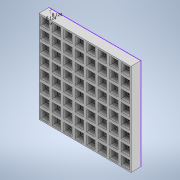
# Autodesk Inventor part: StandMatrix
Saved by Autodesk Inventor 2020.1 (Build 241239000, 239)
## iProperties
Created: 2019-09-02
Part Number: StandMatrix
Material: Generic
Document SubType Name: Modeling
Designer: matteo.spadetto-1
Density: 1 g/cm^3
Appearance: Default
Author: matteo.spadetto-1
Autodesk Inventor part; units mm, degrees
ref_plane "YZ Plane" through (0, 0, 0) normal (1, 0, 0) x (0, 1, 0)
ref_plane "XZ Plane" through (0, 0, 0) normal (0, 1, 0) x (-1, 0, 0)
ref_plane "XY Plane" through (0, 0, 0) normal (0, 0, 1) x (1, 0, 0)
sketch "Sketch1" plane through (0, 0, 0) normal (0, 0, 1) x (1, 0, 0)
  line L0 (1.062, 57.938) -> (1.062, 63.938)
  line L1 (1.062, 63.938) -> (7.062, 63.938)
  line L2 (7.062, 63.938) -> (7.062, 57.938)
  line L3 (7.062, 57.938) -> (1.062, 57.938)
  line L4 (17.31, 57.938) -> (23.31, 57.938)
  line L5 (23.31, 57.938) -> (23.31, 63.938)
  line L6 (23.31, 63.938) -> (17.31, 63.938)
  line L7 (17.31, 63.938) -> (17.31, 57.938)
  line L8 (9.186, 57.938) -> (15.186, 57.938)
  line L9 (15.186, 57.938) -> (15.186, 63.938)
  line L10 (15.186, 63.938) -> (9.186, 63.938)
  line L11 (9.186, 63.938) -> (9.186, 57.938)
  line L12 (25.434, 57.938) -> (31.434, 57.938)
  line L13 (31.434, 57.938) -> (31.434, 63.938)
  line L14 (31.434, 63.938) -> (25.434, 63.938)
  line L15 (25.434, 63.938) -> (25.434, 57.938)
  line L16 (33.558, 57.938) -> (39.558, 57.938)
  line L17 (39.558, 57.938) -> (39.558, 63.938)
  line L18 (39.558, 63.938) -> (33.558, 63.938)
  line L19 (33.558, 63.938) -> (33.558, 57.938)
  line L20 (47.682, 57.938) -> (41.682, 57.938)
  line L21 (41.682, 57.938) -> (41.682, 63.938)
  line L22 (41.682, 63.938) -> (47.682, 63.938)
  line L23 (47.682, 63.938) -> (47.682, 57.938)
  line L24 (55.806, 57.938) -> (49.806, 57.938)
  line L25 (49.806, 57.938) -> (49.806, 63.938)
  line L26 (49.806, 63.938) -> (55.806, 63.938)
  line L27 (55.806, 63.938) -> (55.806, 57.938)
  line L28 (63.93, 57.938) -> (57.93, 57.938)
  line L29 (57.93, 57.938) -> (57.93, 63.938)
  line L30 (57.93, 63.938) -> (63.93, 63.938)
  line L31 (63.93, 63.938) -> (63.93, 57.938)
  line L32 (1.062, 49.814) -> (1.062, 55.814)
  line L33 (1.062, 55.814) -> (7.062, 55.814)
  line L34 (7.062, 55.814) -> (7.062, 49.814)
  line L35 (7.062, 49.814) -> (1.062, 49.814)
  line L36 (9.186, 49.814) -> (15.186, 49.814)
  line L37 (15.186, 49.814) -> (15.186, 55.814)
  line L38 (15.186, 55.814) -> (9.186, 55.814)
  line L39 (9.186, 55.814) -> (9.186, 49.814)
  line L40 (17.31, 49.814) -> (17.31, 55.814)
  line L41 (17.31, 55.814) -> (23.31, 55.814)
  line L42 (23.31, 55.814) -> (23.31, 49.814)
  line L43 (23.31, 49.814) -> (17.31, 49.814)
  line L44 (25.434, 55.814) -> (31.434, 55.814)
  line L45 (31.434, 55.814) -> (31.434, 49.814)
  line L46 (31.434, 49.814) -> (25.434, 49.814)
  line L47 (33.558, 55.814) -> (39.558, 55.814)
  line L48 (39.558, 55.814) -> (39.558, 49.814)
  line L49 (39.558, 49.814) -> (33.558, 49.814)
  line L50 (47.682, 49.814) -> (41.682, 49.814)
  line L51 (41.682, 49.814) -> (41.682, 55.814)
  line L52 (41.682, 55.814) -> (47.682, 55.814)
  line L53 (47.682, 55.814) -> (47.682, 49.814)
  line L54 (49.806, 49.814) -> (55.806, 49.814)
  line L55 (55.806, 49.814) -> (55.806, 55.814)
  line L56 (55.806, 55.814) -> (49.806, 55.814)
  line L57 (49.806, 55.814) -> (49.806, 49.814)
  line L58 (63.93, 49.814) -> (57.93, 49.814)
  line L59 (57.93, 49.814) -> (57.93, 55.814)
  line L60 (57.93, 55.814) -> (63.93, 55.814)
  line L61 (63.93, 55.814) -> (63.93, 49.814)
  line L62 (1.062, 41.69) -> (7.062, 41.69)
  line L63 (7.062, 41.69) -> (7.062, 47.69)
  line L64 (7.062, 47.69) -> (1.062, 47.69)
  line L65 (1.062, 47.69) -> (1.062, 41.69)
  line L66 (9.186, 41.69) -> (9.186, 47.69)
  line L67 (9.186, 47.69) -> (15.186, 47.69)
  line L68 (15.186, 47.69) -> (15.186, 41.69)
  line L69 (15.186, 41.69) -> (9.186, 41.69)
  line L70 (23.31, 41.69) -> (23.31, 47.69)
  line L71 (23.31, 47.69) -> (17.31, 47.69)
  line L72 (17.31, 47.69) -> (17.31, 41.69)
  line L73 (17.31, 41.69) -> (23.31, 41.69)
  line L74 (31.434, 41.69) -> (25.434, 41.69)
  line L75 (25.434, 41.69) -> (25.434, 47.69)
  line L76 (25.434, 47.69) -> (31.434, 47.69)
  line L77 (31.434, 47.69) -> (31.434, 41.69)
  line L78 (39.558, 41.69) -> (33.558, 41.69)
  line L79 (33.558, 41.69) -> (33.558, 47.69)
  line L80 (33.558, 47.69) -> (39.558, 47.69)
  line L81 (39.558, 47.69) -> (39.558, 41.69)
  line L82 (47.682, 41.69) -> (47.682, 47.69)
  line L83 (47.682, 47.69) -> (41.682, 47.69)
  line L84 (41.682, 47.69) -> (41.682, 41.69)
  line L85 (41.682, 41.69) -> (47.682, 41.69)
  line L86 (55.806, 41.69) -> (55.806, 47.69)
  line L87 (55.806, 47.69) -> (49.806, 47.69)
  line L88 (49.806, 47.69) -> (49.806, 41.69)
  line L89 (49.806, 41.69) -> (55.806, 41.69)
  line L90 (63.93, 41.69) -> (63.93, 47.69)
  line L91 (63.93, 47.69) -> (57.93, 47.69)
  line L92 (57.93, 47.69) -> (57.93, 41.69)
  line L93 (57.93, 41.69) -> (63.93, 41.69)
  line L94 (7.062, 33.566) -> (1.062, 33.566)
  line L95 (1.062, 33.566) -> (1.062, 39.566)
  line L96 (1.062, 39.566) -> (7.062, 39.566)
  line L97 (7.062, 39.566) -> (7.062, 33.566)
  line L98 (15.186, 33.566) -> (15.186, 39.566)
  line L99 (15.186, 39.566) -> (9.186, 39.566)
  line L100 (9.186, 39.566) -> (9.186, 33.566)
  line L101 (9.186, 33.566) -> (15.186, 33.566)
  line L102 (17.31, 33.566) -> (23.31, 33.566)
  line L103 (23.31, 33.566) -> (23.31, 39.566)
  line L104 (23.31, 39.566) -> (17.31, 39.566)
  line L105 (17.31, 39.566) -> (17.31, 33.566)
  line L106 (25.434, 33.566) -> (31.434, 33.566)
  line L107 (31.434, 33.566) -> (31.434, 39.566)
  line L108 (31.434, 39.566) -> (25.434, 39.566)
  line L109 (25.434, 39.566) -> (25.434, 33.566)
  line L110 (39.558, 33.566) -> (33.558, 33.566)
  line L111 (33.558, 33.566) -> (33.558, 39.566)
  line L112 (33.558, 39.566) -> (39.558, 39.566)
  line L113 (39.558, 39.566) -> (39.558, 33.566)
  line L114 (41.682, 33.566) -> (41.682, 39.566)
  line L115 (41.682, 39.566) -> (47.682, 39.566)
  line L116 (47.682, 39.566) -> (47.682, 33.566)
  line L117 (47.682, 33.566) -> (41.682, 33.566)
  line L118 (55.806, 33.566) -> (49.806, 33.566)
  line L119 (49.806, 33.566) -> (49.806, 39.566)
  line L120 (49.806, 39.566) -> (55.806, 39.566)
  line L121 (55.806, 39.566) -> (55.806, 33.566)
  line L122 (63.93, 33.566) -> (57.93, 33.566)
  line L123 (57.93, 33.566) -> (57.93, 39.566)
  line L124 (57.93, 39.566) -> (63.93, 39.566)
  line L125 (63.93, 39.566) -> (63.93, 33.566)
  line L126 (25.434, 49.814) -> (25.434, 55.814)
  line L127 (33.558, 55.814) -> (33.558, 49.814)
  line L128 (1.062, 7.062) -> (1.062, 1.062)
  line L129 (1.062, 1.062) -> (7.062, 1.062)
  line L130 (7.062, 1.062) -> (7.062, 7.062)
  line L131 (7.062, 7.062) -> (1.062, 7.062)
  line L132 (17.31, 7.062) -> (23.31, 7.062)
  line L133 (23.31, 7.062) -> (23.31, 1.062)
  line L134 (23.31, 1.062) -> (17.31, 1.062)
  line L135 (17.31, 1.062) -> (17.31, 7.062)
  line L136 (9.186, 7.062) -> (15.186, 7.062)
  line L137 (15.186, 7.062) -> (15.186, 1.062)
  line L138 (15.186, 1.062) -> (9.186, 1.062)
  line L139 (9.186, 1.062) -> (9.186, 7.062)
  line L140 (25.434, 7.062) -> (31.434, 7.062)
  line L141 (31.434, 7.062) -> (31.434, 1.062)
  line L142 (31.434, 1.062) -> (25.434, 1.062)
  line L143 (25.434, 1.062) -> (25.434, 7.062)
  line L144 (33.558, 7.062) -> (39.558, 7.062)
  line L145 (39.558, 7.062) -> (39.558, 1.062)
  line L146 (39.558, 1.062) -> (33.558, 1.062)
  line L147 (33.558, 1.062) -> (33.558, 7.062)
  line L148 (47.682, 7.062) -> (41.682, 7.062)
  line L149 (41.682, 7.062) -> (41.682, 1.062)
  line L150 (41.682, 1.062) -> (47.682, 1.062)
  line L151 (47.682, 1.062) -> (47.682, 7.062)
  line L152 (55.806, 7.062) -> (49.806, 7.062)
  line L153 (49.806, 7.062) -> (49.806, 1.062)
  line L154 (49.806, 1.062) -> (55.806, 1.062)
  line L155 (55.806, 1.062) -> (55.806, 7.062)
  line L156 (63.93, 7.062) -> (57.93, 7.062)
  line L157 (57.93, 7.062) -> (57.93, 1.062)
  line L158 (57.93, 1.062) -> (63.93, 1.062)
  line L159 (63.93, 1.062) -> (63.93, 7.062)
  line L160 (1.062, 15.186) -> (1.062, 9.186)
  line L161 (1.062, 9.186) -> (7.062, 9.186)
  line L162 (7.062, 9.186) -> (7.062, 15.186)
  line L163 (7.062, 15.186) -> (1.062, 15.186)
  line L164 (9.186, 15.186) -> (15.186, 15.186)
  line L165 (15.186, 15.186) -> (15.186, 9.186)
  line L166 (15.186, 9.186) -> (9.186, 9.186)
  line L167 (9.186, 9.186) -> (9.186, 15.186)
  line L168 (17.31, 15.186) -> (17.31, 9.186)
  line L169 (17.31, 9.186) -> (23.31, 9.186)
  line L170 (23.31, 9.186) -> (23.31, 15.186)
  line L171 (23.31, 15.186) -> (17.31, 15.186)
  line L172 (25.434, 9.186) -> (31.434, 9.186)
  line L173 (31.434, 9.186) -> (31.434, 15.186)
  line L174 (31.434, 15.186) -> (25.434, 15.186)
  line L175 (33.558, 9.186) -> (39.558, 9.186)
  line L176 (39.558, 9.186) -> (39.558, 15.186)
  line L177 (39.558, 15.186) -> (33.558, 15.186)
  line L178 (47.682, 15.186) -> (41.682, 15.186)
  line L179 (41.682, 15.186) -> (41.682, 9.186)
  line L180 (41.682, 9.186) -> (47.682, 9.186)
  line L181 (47.682, 9.186) -> (47.682, 15.186)
  line L182 (49.806, 15.186) -> (55.806, 15.186)
  line L183 (55.806, 15.186) -> (55.806, 9.186)
  line L184 (55.806, 9.186) -> (49.806, 9.186)
  line L185 (49.806, 9.186) -> (49.806, 15.186)
  line L186 (63.93, 15.186) -> (57.93, 15.186)
  line L187 (57.93, 15.186) -> (57.93, 9.186)
  line L188 (57.93, 9.186) -> (63.93, 9.186)
  line L189 (63.93, 9.186) -> (63.93, 15.186)
  line L190 (1.062, 23.31) -> (7.062, 23.31)
  line L191 (7.062, 23.31) -> (7.062, 17.31)
  line L192 (7.062, 17.31) -> (1.062, 17.31)
  line L193 (1.062, 17.31) -> (1.062, 23.31)
  line L194 (9.186, 23.31) -> (9.186, 17.31)
  line L195 (9.186, 17.31) -> (15.186, 17.31)
  line L196 (15.186, 17.31) -> (15.186, 23.31)
  line L197 (15.186, 23.31) -> (9.186, 23.31)
  line L198 (23.31, 23.31) -> (23.31, 17.31)
  line L199 (23.31, 17.31) -> (17.31, 17.31)
  line L200 (17.31, 17.31) -> (17.31, 23.31)
  line L201 (17.31, 23.31) -> (23.31, 23.31)
  line L202 (31.434, 23.31) -> (25.434, 23.31)
  line L203 (25.434, 23.31) -> (25.434, 17.31)
  line L204 (25.434, 17.31) -> (31.434, 17.31)
  line L205 (31.434, 17.31) -> (31.434, 23.31)
  line L206 (39.558, 23.31) -> (33.558, 23.31)
  line L207 (33.558, 23.31) -> (33.558, 17.31)
  line L208 (33.558, 17.31) -> (39.558, 17.31)
  line L209 (39.558, 17.31) -> (39.558, 23.31)
  line L210 (47.682, 23.31) -> (47.682, 17.31)
  line L211 (47.682, 17.31) -> (41.682, 17.31)
  line L212 (41.682, 17.31) -> (41.682, 23.31)
  line L213 (41.682, 23.31) -> (47.682, 23.31)
  line L214 (55.806, 23.31) -> (55.806, 17.31)
  line L215 (55.806, 17.31) -> (49.806, 17.31)
  line L216 (49.806, 17.31) -> (49.806, 23.31)
  line L217 (49.806, 23.31) -> (55.806, 23.31)
  line L218 (63.93, 23.31) -> (63.93, 17.31)
  line L219 (63.93, 17.31) -> (57.93, 17.31)
  line L220 (57.93, 17.31) -> (57.93, 23.31)
  line L221 (57.93, 23.31) -> (63.93, 23.31)
  line L222 (7.062, 31.434) -> (1.062, 31.434)
  line L223 (1.062, 31.434) -> (1.062, 25.434)
  line L224 (1.062, 25.434) -> (7.062, 25.434)
  line L225 (7.062, 25.434) -> (7.062, 31.434)
  line L226 (15.186, 31.434) -> (15.186, 25.434)
  line L227 (15.186, 25.434) -> (9.186, 25.434)
  line L228 (9.186, 25.434) -> (9.186, 31.434)
  line L229 (9.186, 31.434) -> (15.186, 31.434)
  line L230 (17.31, 31.434) -> (23.31, 31.434)
  line L231 (23.31, 31.434) -> (23.31, 25.434)
  line L232 (23.31, 25.434) -> (17.31, 25.434)
  line L233 (17.31, 25.434) -> (17.31, 31.434)
  line L234 (25.434, 31.434) -> (31.434, 31.434)
  line L235 (31.434, 31.434) -> (31.434, 25.434)
  line L236 (31.434, 25.434) -> (25.434, 25.434)
  line L237 (25.434, 25.434) -> (25.434, 31.434)
  line L238 (39.558, 31.434) -> (33.558, 31.434)
  line L239 (33.558, 31.434) -> (33.558, 25.434)
  line L240 (33.558, 25.434) -> (39.558, 25.434)
  line L241 (39.558, 25.434) -> (39.558, 31.434)
  line L242 (41.682, 31.434) -> (41.682, 25.434)
  line L243 (41.682, 25.434) -> (47.682, 25.434)
  line L244 (47.682, 25.434) -> (47.682, 31.434)
  line L245 (47.682, 31.434) -> (41.682, 31.434)
  line L246 (55.806, 31.434) -> (49.806, 31.434)
  line L247 (49.806, 31.434) -> (49.806, 25.434)
  line L248 (49.806, 25.434) -> (55.806, 25.434)
  line L249 (55.806, 25.434) -> (55.806, 31.434)
  line L250 (63.93, 31.434) -> (57.93, 31.434)
  line L251 (57.93, 31.434) -> (57.93, 25.434)
  line L252 (57.93, 25.434) -> (63.93, 25.434)
  line L253 (63.93, 25.434) -> (63.93, 31.434)
  line L254 (25.434, 15.186) -> (25.434, 9.186)
  line L255 (33.558, 9.186) -> (33.558, 15.186)
  line L256 (0, 65) -> (0, 0)
  line L257 (0, 0) -> (65, 0)
  line L258 (0, 65) -> (65, 65)
  line L259 (65, 65) -> (65, 0)
  line L260 (6.562, 63.438) -> (6.562, 58.438)
  line L261 (6.562, 58.438) -> (1.562, 58.438)
  line L262 (1.562, 58.438) -> (1.562, 63.438)
  line L263 (1.562, 63.438) -> (6.562, 63.438)
  line L264 (9.686, 63.438) -> (14.686, 63.438)
  line L265 (14.686, 63.438) -> (14.686, 58.438)
  line L266 (14.686, 58.438) -> (9.686, 58.438)
  line L267 (9.686, 58.438) -> (9.686, 63.438)
  line L268 (17.81, 63.438) -> (22.81, 63.438)
  line L269 (22.81, 63.438) -> (22.81, 58.438)
  line L270 (22.81, 58.438) -> (17.81, 58.438)
  line L271 (17.81, 58.438) -> (17.81, 63.438)
  line L272 (25.934, 63.438) -> (30.934, 63.438)
  line L273 (30.934, 63.438) -> (30.934, 58.438)
  line L274 (30.934, 58.438) -> (25.934, 58.438)
  line L275 (25.934, 58.438) -> (25.934, 63.438)
  line L276 (34.058, 63.438) -> (39.058, 63.438)
  line L277 (39.058, 63.438) -> (39.058, 58.438)
  line L278 (39.058, 58.438) -> (34.058, 58.438)
  line L279 (34.058, 58.438) -> (34.058, 63.438)
  line L280 (42.182, 63.438) -> (47.182, 63.438)
  line L281 (47.182, 63.438) -> (47.182, 58.438)
  line L282 (47.182, 58.438) -> (42.182, 58.438)
  line L283 (42.182, 58.438) -> (42.182, 63.438)
  line L284 (50.306, 63.438) -> (55.306, 63.438)
  line L285 (55.306, 63.438) -> (55.306, 58.438)
  line L286 (55.306, 58.438) -> (50.306, 58.438)
  line L287 (50.306, 58.438) -> (50.306, 63.438)
  line L288 (58.43, 63.438) -> (63.43, 63.438)
  line L289 (63.43, 63.438) -> (63.43, 58.438)
  line L290 (63.43, 58.438) -> (58.43, 58.438)
  line L291 (58.43, 58.438) -> (58.43, 63.438)
  line L292 (1.562, 55.314) -> (6.562, 55.314)
  line L293 (6.562, 55.314) -> (6.562, 50.314)
  line L294 (6.562, 50.314) -> (1.562, 50.314)
  line L295 (1.562, 50.314) -> (1.562, 55.314)
  line L296 (9.686, 55.314) -> (14.686, 55.314)
  line L297 (14.686, 55.314) -> (14.686, 50.314)
  line L298 (14.686, 50.314) -> (9.686, 50.314)
  line L299 (9.686, 50.314) -> (9.686, 55.314)
  line L300 (17.81, 55.314) -> (22.81, 55.314)
  line L301 (22.81, 55.314) -> (22.81, 50.314)
  line L302 (22.81, 50.314) -> (17.81, 50.314)
  line L303 (17.81, 50.314) -> (17.81, 55.314)
  line L304 (25.934, 55.314) -> (30.934, 55.314)
  line L305 (30.934, 55.314) -> (30.934, 50.314)
  line L306 (30.934, 50.314) -> (25.934, 50.314)
  line L307 (25.934, 50.314) -> (25.934, 55.314)
  line L308 (34.058, 55.314) -> (39.058, 55.314)
  line L309 (39.058, 55.314) -> (39.058, 50.314)
  line L310 (39.058, 50.314) -> (34.058, 50.314)
  line L311 (34.058, 50.314) -> (34.058, 55.314)
  line L312 (42.182, 55.314) -> (47.182, 55.314)
  line L313 (47.182, 55.314) -> (47.182, 50.314)
  line L314 (47.182, 50.314) -> (42.182, 50.314)
  line L315 (42.182, 50.314) -> (42.182, 55.314)
  line L316 (50.306, 55.314) -> (55.306, 55.314)
  line L317 (55.306, 55.314) -> (55.306, 50.314)
  line L318 (55.306, 50.314) -> (50.306, 50.314)
  line L319 (50.306, 50.314) -> (50.306, 55.314)
  line L320 (58.43, 55.314) -> (63.43, 55.314)
  line L321 (63.43, 55.314) -> (63.43, 50.314)
  line L322 (63.43, 50.314) -> (58.43, 50.314)
  line L323 (58.43, 50.314) -> (58.43, 55.314)
  line L324 (1.562, 47.19) -> (6.562, 47.19)
  line L325 (6.562, 47.19) -> (6.562, 42.19)
  line L326 (6.562, 42.19) -> (1.562, 42.19)
  line L327 (1.562, 42.19) -> (1.562, 47.19)
  line L328 (9.686, 47.19) -> (14.686, 47.19)
  line L329 (14.686, 47.19) -> (14.686, 42.19)
  line L330 (14.686, 42.19) -> (9.686, 42.19)
  line L331 (9.686, 42.19) -> (9.686, 47.19)
  line L332 (17.81, 47.19) -> (22.81, 47.19)
  line L333 (22.81, 47.19) -> (22.81, 42.19)
  line L334 (22.81, 42.19) -> (17.81, 42.19)
  line L335 (17.81, 42.19) -> (17.81, 47.19)
  line L336 (25.934, 47.19) -> (30.934, 47.19)
  line L337 (30.934, 47.19) -> (30.934, 42.19)
  line L338 (30.934, 42.19) -> (25.934, 42.19)
  line L339 (25.934, 42.19) -> (25.934, 47.19)
  line L340 (34.058, 47.19) -> (39.058, 47.19)
  line L341 (39.058, 47.19) -> (39.058, 42.19)
  line L342 (39.058, 42.19) -> (34.058, 42.19)
  line L343 (34.058, 42.19) -> (34.058, 47.19)
  line L344 (42.182, 47.19) -> (47.182, 47.19)
  line L345 (47.182, 47.19) -> (47.182, 42.19)
  line L346 (47.182, 42.19) -> (42.182, 42.19)
  line L347 (42.182, 42.19) -> (42.182, 47.19)
  line L348 (50.306, 47.19) -> (55.306, 47.19)
  line L349 (55.306, 47.19) -> (55.306, 42.19)
  line L350 (55.306, 42.19) -> (50.306, 42.19)
  line L351 (50.306, 42.19) -> (50.306, 47.19)
  line L352 (58.43, 47.19) -> (63.43, 47.19)
  line L353 (63.43, 47.19) -> (63.43, 42.19)
  line L354 (63.43, 42.19) -> (58.43, 42.19)
  line L355 (58.43, 42.19) -> (58.43, 47.19)
  line L356 (1.562, 39.066) -> (6.562, 39.066)
  line L357 (6.562, 39.066) -> (6.562, 34.066)
  line L358 (6.562, 34.066) -> (1.562, 34.066)
  line L359 (1.562, 34.066) -> (1.562, 39.066)
  line L360 (9.686, 39.066) -> (14.686, 39.066)
  line L361 (14.686, 39.066) -> (14.686, 34.066)
  line L362 (14.686, 34.066) -> (9.686, 34.066)
  line L363 (9.686, 34.066) -> (9.686, 39.066)
  line L364 (17.81, 39.066) -> (22.81, 39.066)
  line L365 (22.81, 39.066) -> (22.81, 34.066)
  line L366 (22.81, 34.066) -> (17.81, 34.066)
  line L367 (17.81, 34.066) -> (17.81, 39.066)
  line L368 (25.934, 39.066) -> (30.934, 39.066)
  line L369 (30.934, 39.066) -> (30.934, 34.066)
  line L370 (30.934, 34.066) -> (25.934, 34.066)
  line L371 (25.934, 34.066) -> (25.934, 39.066)
  line L372 (34.058, 39.066) -> (39.058, 39.066)
  line L373 (39.058, 39.066) -> (39.058, 34.066)
  line L374 (39.058, 34.066) -> (34.058, 34.066)
  line L375 (34.058, 34.066) -> (34.058, 39.066)
  line L376 (42.182, 39.066) -> (47.182, 39.066)
  line L377 (47.182, 39.066) -> (47.182, 34.066)
  line L378 (47.182, 34.066) -> (42.182, 34.066)
  line L379 (42.182, 34.066) -> (42.182, 39.066)
  line L380 (50.306, 39.066) -> (55.306, 39.066)
  line L381 (55.306, 39.066) -> (55.306, 34.066)
  line L382 (55.306, 34.066) -> (50.306, 34.066)
  line L383 (50.306, 34.066) -> (50.306, 39.066)
  line L384 (58.43, 39.066) -> (63.43, 39.066)
  line L385 (63.43, 39.066) -> (63.43, 34.066)
  line L386 (63.43, 34.066) -> (58.43, 34.066)
  line L387 (58.43, 34.066) -> (58.43, 39.066)
  line L388 (1.562, 30.942) -> (6.562, 30.942)
  line L389 (6.562, 30.942) -> (6.562, 25.942)
  line L390 (6.562, 25.942) -> (1.562, 25.942)
  line L391 (1.562, 25.942) -> (1.562, 30.942)
  line L392 (9.686, 30.942) -> (14.686, 30.942)
  line L393 (14.686, 30.942) -> (14.686, 25.942)
  line L394 (14.686, 25.942) -> (9.686, 25.942)
  line L395 (9.686, 25.942) -> (9.686, 30.942)
  line L396 (17.81, 30.942) -> (22.81, 30.942)
  line L397 (22.81, 30.942) -> (22.81, 25.942)
  line L398 (22.81, 25.942) -> (17.81, 25.942)
  line L399 (17.81, 25.942) -> (17.81, 30.942)
  line L400 (25.934, 30.942) -> (30.934, 30.942)
  line L401 (30.934, 30.942) -> (30.934, 25.942)
  line L402 (30.934, 25.942) -> (25.934, 25.942)
  line L403 (25.934, 25.942) -> (25.934, 30.942)
  line L404 (34.058, 30.942) -> (39.058, 30.942)
  line L405 (39.058, 30.942) -> (39.058, 25.942)
  line L406 (39.058, 25.942) -> (34.058, 25.942)
  line L407 (34.058, 25.942) -> (34.058, 30.942)
  line L408 (42.182, 30.942) -> (47.182, 30.942)
  line L409 (47.182, 30.942) -> (47.182, 25.942)
  line L410 (47.182, 25.942) -> (42.182, 25.942)
  line L411 (42.182, 25.942) -> (42.182, 30.942)
  line L412 (50.306, 30.942) -> (55.306, 30.942)
  line L413 (55.306, 30.942) -> (55.306, 25.942)
  line L414 (55.306, 25.942) -> (50.306, 25.942)
  line L415 (50.306, 25.942) -> (50.306, 30.942)
  line L416 (58.43, 30.942) -> (63.43, 30.942)
  line L417 (63.43, 30.942) -> (63.43, 25.942)
  line L418 (63.43, 25.942) -> (58.43, 25.942)
  line L419 (58.43, 25.942) -> (58.43, 30.942)
  line L420 (1.562, 22.818) -> (6.562, 22.818)
  line L421 (6.562, 22.818) -> (6.562, 17.818)
  line L422 (6.562, 17.818) -> (1.562, 17.818)
  line L423 (1.562, 17.818) -> (1.562, 22.818)
  line L424 (9.686, 22.818) -> (14.686, 22.818)
  line L425 (14.686, 22.818) -> (14.686, 17.818)
  line L426 (14.686, 17.818) -> (9.686, 17.818)
  line L427 (9.686, 17.818) -> (9.686, 22.818)
  line L428 (17.81, 22.818) -> (22.81, 22.818)
  line L429 (22.81, 22.818) -> (22.81, 17.818)
  line L430 (22.81, 17.818) -> (17.81, 17.818)
  line L431 (17.81, 17.818) -> (17.81, 22.818)
  line L432 (25.934, 22.818) -> (30.934, 22.818)
  line L433 (30.934, 22.818) -> (30.934, 17.818)
  line L434 (30.934, 17.818) -> (25.934, 17.818)
  line L435 (25.934, 17.818) -> (25.934, 22.818)
  line L436 (34.058, 22.818) -> (39.058, 22.818)
  line L437 (39.058, 22.818) -> (39.058, 17.818)
  line L438 (39.058, 17.818) -> (34.058, 17.818)
  line L439 (34.058, 17.818) -> (34.058, 22.818)
  line L440 (42.182, 22.818) -> (47.182, 22.818)
  line L441 (47.182, 22.818) -> (47.182, 17.818)
  line L442 (47.182, 17.818) -> (42.182, 17.818)
  line L443 (42.182, 17.818) -> (42.182, 22.818)
  line L444 (50.306, 22.818) -> (55.306, 22.818)
  line L445 (55.306, 22.818) -> (55.306, 17.818)
  line L446 (55.306, 17.818) -> (50.306, 17.818)
  line L447 (50.306, 17.818) -> (50.306, 22.818)
  line L448 (58.43, 22.818) -> (63.43, 22.818)
  line L449 (63.43, 22.818) -> (63.43, 17.818)
  line L450 (63.43, 17.818) -> (58.43, 17.818)
  line L451 (58.43, 17.818) -> (58.43, 22.818)
  line L452 (1.562, 14.694) -> (6.562, 14.694)
  line L453 (6.562, 14.694) -> (6.562, 9.694)
  line L454 (6.562, 9.694) -> (1.562, 9.694)
  line L455 (1.562, 9.694) -> (1.562, 14.694)
  line L456 (9.686, 14.694) -> (14.686, 14.694)
  line L457 (14.686, 14.694) -> (14.686, 9.694)
  line L458 (14.686, 9.694) -> (9.686, 9.694)
  line L459 (9.686, 9.694) -> (9.686, 14.694)
  line L460 (17.81, 14.694) -> (22.81, 14.694)
  line L461 (22.81, 14.694) -> (22.81, 9.694)
  line L462 (22.81, 9.694) -> (17.81, 9.694)
  line L463 (17.81, 9.694) -> (17.81, 14.694)
  line L464 (25.934, 14.694) -> (30.934, 14.694)
  line L465 (30.934, 14.694) -> (30.934, 9.694)
  line L466 (30.934, 9.694) -> (25.934, 9.694)
  line L467 (25.934, 9.694) -> (25.934, 14.694)
  line L468 (34.058, 14.694) -> (39.058, 14.694)
  line L469 (39.058, 14.694) -> (39.058, 9.694)
  line L470 (39.058, 9.694) -> (34.058, 9.694)
  line L471 (34.058, 9.694) -> (34.058, 14.694)
  line L472 (42.182, 14.694) -> (47.182, 14.694)
  line L473 (47.182, 14.694) -> (47.182, 9.694)
  line L474 (47.182, 9.694) -> (42.182, 9.694)
  line L475 (42.182, 9.694) -> (42.182, 14.694)
  line L476 (50.306, 14.694) -> (55.306, 14.694)
  line L477 (55.306, 14.694) -> (55.306, 9.694)
  line L478 (55.306, 9.694) -> (50.306, 9.694)
  line L479 (50.306, 9.694) -> (50.306, 14.694)
  line L480 (58.43, 14.694) -> (63.43, 14.694)
  line L481 (63.43, 14.694) -> (63.43, 9.694)
  line L482 (63.43, 9.694) -> (58.43, 9.694)
  line L483 (58.43, 9.694) -> (58.43, 14.694)
  line L484 (1.562, 6.57) -> (6.562, 6.57)
  line L485 (6.562, 6.57) -> (6.562, 1.57)
  line L486 (6.562, 1.57) -> (1.562, 1.57)
  line L487 (1.562, 1.57) -> (1.562, 6.57)
  line L488 (9.686, 6.57) -> (14.686, 6.57)
  line L489 (14.686, 6.57) -> (14.686, 1.57)
  line L490 (14.686, 1.57) -> (9.686, 1.57)
  line L491 (9.686, 1.57) -> (9.686, 6.57)
  line L492 (17.81, 6.57) -> (22.81, 6.57)
  line L493 (22.81, 6.57) -> (22.81, 1.57)
  line L494 (22.81, 1.57) -> (17.81, 1.57)
  line L495 (17.81, 1.57) -> (17.81, 6.57)
  line L496 (25.934, 6.57) -> (30.934, 6.57)
  line L497 (30.934, 6.57) -> (30.934, 1.57)
  line L498 (30.934, 1.57) -> (25.934, 1.57)
  line L499 (25.934, 1.57) -> (25.934, 6.57)
  line L500 (34.058, 6.57) -> (39.058, 6.57)
  line L501 (39.058, 6.57) -> (39.058, 1.57)
  line L502 (39.058, 1.57) -> (34.058, 1.57)
  line L503 (34.058, 1.57) -> (34.058, 6.57)
  line L504 (42.182, 6.57) -> (47.182, 6.57)
  line L505 (47.182, 6.57) -> (47.182, 1.57)
  line L506 (47.182, 1.57) -> (42.182, 1.57)
  line L507 (42.182, 1.57) -> (42.182, 6.57)
  line L508 (50.306, 6.57) -> (55.306, 6.57)
  line L509 (55.306, 6.57) -> (55.306, 1.57)
  line L510 (55.306, 1.57) -> (50.306, 1.57)
  line L511 (50.306, 1.57) -> (50.306, 6.57)
  line L512 (58.43, 6.57) -> (63.43, 6.57)
  line L513 (63.43, 6.57) -> (63.43, 1.57)
  line L514 (63.43, 1.57) -> (58.43, 1.57)
  line L515 (58.43, 1.57) -> (58.43, 6.57)
  dimension "d70" = 8.124
  dimension "d73" = 8.124
  constraints: 1032 end point, 2 collinear, 1 horizontal, 1 parallel, 1 vertical, 502 other
  measures "d70" distance of L262.end L264.start
  measures "d73" distance of L262.end L292.start
extrude "Extrusion1" add sketch "Sketch1" along normal blind 7 contours L258 L259 L257 L256
extrude "Extrusion2" add sketch "Sketch1" along normal blind 3.5 contours L0 L1 L2 L3 | L7 L6 L5 L4 | L11 L10 L9 L8 | L15 L14 L13 L12 | L19 L18 L17 L16 | L20 L21 L22 L23 | L24 L25 L26 L27 | L28 L29 L30 L31 | L32 L33 L34 L35 | L39 L38 L37 L36 | L40 L41 L42 L43 | L44 L45 L46 L126 | L47 L48 L49 L127 | L50 L51 L52 L53 | L57 L56 L55 L54 | L58 L59 L60 L61 | L65 L64 L63 L62 | L66 L67 L68 L69 | L73 L72 L71 L70 | L74 L75 L76 L77 | L78 L79 L80 L81 | L85 L84 L83 L82 | L89 L88 L87 L86 | L93 L92 L91 L90 | L94 L95 L96 L97 | L101 L100 L99 L98 | L105 L104 L103 L102 | L109 L108 L107 L106 | L110 L111 L112 L113 | L114 L115 L116 L117 | L118 L119 L120 L121 | L122 L123 L124 L125 | L131 L130 L129 L128 | L132 L133 L134 L135 | L136 L137 L138 L139 | L140 L141 L142 L143 | L144 L145 L146 L147 | L151 L150 L149 L148 | L155 L154 L153 L152 | L159 L158 L157 L156 | L163 L162 L161 L160 | L164 L165 L166 L167 | L171 L170 L169 L168 | L254 L174 L173 L172 | L255 L177 L176 L175 | L181 L180 L179 L178 | L182 L183 L184 L185 | L189 L188 L187 L186 | L190 L191 L192 L193 | L197 L196 L195 L194 | L198 L199 L200 L201 | L205 L204 L203 L202 | L209 L208 L207 L206 | L210 L211 L212 L213 | L214 L215 L216 L217 | L218 L219 L220 L221 | L225 L224 L223 L222 | L226 L227 L228 L229 | L230 L231 L232 L233 | L234 L235 L236 L237 | L241 L240 L239 L238 | L245 L244 L243 L242 | L249 L248 L247 L246 | L253 L252 L251 L250 | L258 L259 L257 L256 | L260 L261 L262 L263 | L264 L265 L266 L267 | L268 L269 L270 L271 | L272 L273 L274 L275 | L276 L277 L278 L279 | L280 L281 L282 L283 | L284 L285 L286 L287 | L288 L289 L290 L291 | L292 L293 L294 L295 | L296 L297 L298 L299 | L300 L301 L302 L303 | L304 L305 L306 L307 | L308 L309 L310 L311 | L312 L313 L314 L315 | L316 L317 L318 L319 | L320 L321 L322 L323 | L324 L325 L326 L327 | L328 L329 L330 L331 | L332 L333 L334 L335 | L336 L337 L338 L339 | L340 L341 L342 L343 | L344 L345 L346 L347 | L348 L349 L350 L351 | L352 L353 L354 L355 | L356 L357 L358 L359 | L360 L361 L362 L363 | L364 L365 L366 L367 | L368 L369 L370 L371 | L372 L373 L374 L375 | L376 L377 L378 L379 | L380 L381 L382 L383 | L384 L385 L386 L387 | L388 L389 L390 L391 | L392 L393 L394 L395 | L396 L397 L398 L399 | L400 L401 L402 L403 | L404 L405 L406 L407 | L408 L409 L410 L411 | L412 L413 L414 L415 | L416 L417 L418 L419 | L420 L421 L422 L423 | L424 L425 L426 L427 | L428 L429 L430 L431 | L432 L433 L434 L435 | L436 L437 L438 L439 | L440 L441 L442 L443 | L444 L445 L446 L447 | L448 L449 L450 L451 | L452 L453 L454 L455 | L456 L457 L458 L459 | L460 L461 L462 L463 | L464 L465 L466 L467 | L468 L469 L470 L471 | L472 L473 L474 L475 | L476 L477 L478 L479 | L480 L481 L482 L483 | L484 L485 L486 L487 | L488 L489 L490 L491 | L492 L493 L494 L495 | L496 L497 L498 L499 | L500 L501 L502 L503 | L504 L505 L506 L507 | L508 L509 L510 L511 | L512 L513 L514 L515
extrude "Extrusion4" cut sketch "Sketch1" along normal blind 2.5 contours L0 L1 L2 L3 | L7 L6 L5 L4 | L11 L10 L9 L8 | L15 L14 L13 L12 | L19 L18 L17 L16 | L20 L21 L22 L23 | L24 L25 L26 L27 | L28 L29 L30 L31 | L32 L33 L34 L35 | L39 L38 L37 L36 | L40 L41 L42 L43 | L44 L45 L46 L126 | L47 L48 L49 L127 | L50 L51 L52 L53 | L57 L56 L55 L54 | L58 L59 L60 L61 | L65 L64 L63 L62 | L66 L67 L68 L69 | L73 L72 L71 L70 | L74 L75 L76 L77 | L78 L79 L80 L81 | L85 L84 L83 L82 | L89 L88 L87 L86 | L93 L92 L91 L90 | L94 L95 L96 L97 | L101 L100 L99 L98 | L105 L104 L103 L102 | L109 L108 L107 L106 | L110 L111 L112 L113 | L114 L115 L116 L117 | L118 L119 L120 L121 | L122 L123 L124 L125 | L131 L130 L129 L128 | L132 L133 L134 L135 | L136 L137 L138 L139 | L140 L141 L142 L143 | L144 L145 L146 L147 | L151 L150 L149 L148 | L155 L154 L153 L152 | L159 L158 L157 L156 | L163 L162 L161 L160 | L164 L165 L166 L167 | L171 L170 L169 L168 | L254 L174 L173 L172 | L255 L177 L176 L175 | L181 L180 L179 L178 | L182 L183 L184 L185 | L189 L188 L187 L186 | L190 L191 L192 L193 | L197 L196 L195 L194 | L198 L199 L200 L201 | L205 L204 L203 L202 | L209 L208 L207 L206 | L210 L211 L212 L213 | L214 L215 L216 L217 | L218 L219 L220 L221 | L225 L224 L223 L222 | L226 L227 L228 L229 | L230 L231 L232 L233 | L234 L235 L236 L237 | L241 L240 L239 L238 | L245 L244 L243 L242 | L249 L248 L247 L246 | L253 L252 L251 L250 | L260 L261 L262 L263 | L264 L265 L266 L267 | L268 L269 L270 L271 | L272 L273 L274 L275 | L276 L277 L278 L279 | L280 L281 L282 L283 | L284 L285 L286 L287 | L288 L289 L290 L291 | L292 L293 L294 L295 | L296 L297 L298 L299 | L300 L301 L302 L303 | L304 L305 L306 L307 | L308 L309 L310 L311 | L312 L313 L314 L315 | L316 L317 L318 L319 | L320 L321 L322 L323 | L324 L325 L326 L327 | L328 L329 L330 L331 | L332 L333 L334 L335 | L336 L337 L338 L339 | L340 L341 L342 L343 | L344 L345 L346 L347 | L348 L349 L350 L351 | L352 L353 L354 L355 | L356 L357 L358 L359 | L360 L361 L362 L363 | L364 L365 L366 L367 | L368 L369 L370 L371 | L372 L373 L374 L375 | L376 L377 L378 L379 | L380 L381 L382 L383 | L384 L385 L386 L387 | L388 L389 L390 L391 | L392 L393 L394 L395 | L396 L397 L398 L399 | L400 L401 L402 L403 | L404 L405 L406 L407 | L408 L409 L410 L411 | L412 L413 L414 L415 | L416 L417 L418 L419 | L420 L421 L422 L423 | L424 L425 L426 L427 | L428 L429 L430 L431 | L432 L433 L434 L435 | L436 L437 L438 L439 | L440 L441 L442 L443 | L444 L445 L446 L447 | L448 L449 L450 L451 | L452 L453 L454 L455 | L456 L457 L458 L459 | L460 L461 L462 L463 | L464 L465 L466 L467 | L468 L469 L470 L471 | L472 L473 L474 L475 | L476 L477 L478 L479 | L480 L481 L482 L483 | L484 L485 L486 L487 | L488 L489 L490 L491 | L492 L493 L494 L495 | L496 L497 L498 L499 | L500 L501 L502 L503 | L504 L505 L506 L507 | L508 L509 L510 L511 | L512 L513 L514 L515
sketch "Sketch3" plane through (0, 0, 0) normal (0, 0, -1) x (-1, 0, 0)
  line L0 (-57.93, 7.062) -> (-63.93, 7.062)
  line L1 (-63.93, 7.062) -> (-63.93, 1.062)
  line L2 (-58.43, 1.562) -> (-63.43, 1.562)
  line L3 (-63.43, 1.562) -> (-63.43, 6.562)
  line L4 (-63.43, 6.562) -> (-58.43, 6.562)
  line L5 (-58.43, 6.562) -> (-58.43, 1.562)
  line L6 (-58.43, 9.686) -> (-63.43, 9.686)
  line L7 (-63.43, 9.686) -> (-63.43, 14.686)
  line L8 (-63.43, 14.686) -> (-58.43, 14.686)
  line L9 (-58.43, 14.686) -> (-58.43, 9.686)
  line L10 (-58.43, 17.81) -> (-63.43, 17.81)
  line L11 (-63.43, 17.81) -> (-63.43, 22.81)
  line L12 (-63.43, 22.81) -> (-58.43, 22.81)
  line L13 (-58.43, 22.81) -> (-58.43, 17.81)
  line L14 (-58.43, 25.934) -> (-63.43, 25.934)
  line L15 (-63.43, 25.934) -> (-63.43, 30.934)
  line L16 (-63.43, 30.934) -> (-58.43, 30.934)
  line L17 (-58.43, 30.934) -> (-58.43, 25.934)
  line L18 (-58.43, 34.058) -> (-63.43, 34.058)
  line L19 (-63.43, 34.058) -> (-63.43, 39.058)
  line L20 (-63.43, 39.058) -> (-58.43, 39.058)
  line L21 (-58.43, 39.058) -> (-58.43, 34.058)
  line L22 (-58.43, 42.182) -> (-63.43, 42.182)
  line L23 (-63.43, 42.182) -> (-63.43, 47.182)
  line L24 (-63.43, 47.182) -> (-58.43, 47.182)
  line L25 (-58.43, 47.182) -> (-58.43, 42.182)
  line L26 (-58.43, 50.306) -> (-63.43, 50.306)
  line L27 (-63.43, 50.306) -> (-63.43, 55.306)
  line L28 (-63.43, 55.306) -> (-58.43, 55.306)
  line L29 (-58.43, 55.306) -> (-58.43, 50.306)
  line L30 (-58.43, 58.43) -> (-63.43, 58.43)
  line L31 (-63.43, 58.43) -> (-63.43, 63.43)
  line L32 (-63.43, 63.43) -> (-58.43, 63.43)
  line L33 (-58.43, 63.43) -> (-58.43, 58.43)
  line L34 (-50.306, 1.562) -> (-55.306, 1.562)
  line L35 (-55.306, 1.562) -> (-55.306, 6.562)
  line L36 (-55.306, 6.562) -> (-50.306, 6.562)
  line L37 (-50.306, 6.562) -> (-50.306, 1.562)
  line L38 (-50.306, 9.686) -> (-55.306, 9.686)
  line L39 (-55.306, 9.686) -> (-55.306, 14.686)
  line L40 (-55.306, 14.686) -> (-50.306, 14.686)
  line L41 (-50.306, 14.686) -> (-50.306, 9.686)
  line L42 (-50.306, 17.81) -> (-55.306, 17.81)
  line L43 (-55.306, 17.81) -> (-55.306, 22.81)
  line L44 (-55.306, 22.81) -> (-50.306, 22.81)
  line L45 (-50.306, 22.81) -> (-50.306, 17.81)
  line L46 (-50.306, 25.934) -> (-55.306, 25.934)
  line L47 (-55.306, 25.934) -> (-55.306, 30.934)
  line L48 (-55.306, 30.934) -> (-50.306, 30.934)
  line L49 (-50.306, 30.934) -> (-50.306, 25.934)
  line L50 (-50.306, 34.058) -> (-55.306, 34.058)
  line L51 (-55.306, 34.058) -> (-55.306, 39.058)
  line L52 (-55.306, 39.058) -> (-50.306, 39.058)
  line L53 (-50.306, 39.058) -> (-50.306, 34.058)
  line L54 (-50.306, 42.182) -> (-55.306, 42.182)
  line L55 (-55.306, 42.182) -> (-55.306, 47.182)
  line L56 (-55.306, 47.182) -> (-50.306, 47.182)
  line L57 (-50.306, 47.182) -> (-50.306, 42.182)
  line L58 (-50.306, 50.306) -> (-55.306, 50.306)
  line L59 (-55.306, 50.306) -> (-55.306, 55.306)
  line L60 (-55.306, 55.306) -> (-50.306, 55.306)
  line L61 (-50.306, 55.306) -> (-50.306, 50.306)
  line L62 (-50.306, 58.43) -> (-55.306, 58.43)
  line L63 (-55.306, 58.43) -> (-55.306, 63.43)
  line L64 (-55.306, 63.43) -> (-50.306, 63.43)
  line L65 (-50.306, 63.43) -> (-50.306, 58.43)
  line L66 (-42.182, 1.562) -> (-47.182, 1.562)
  line L67 (-47.182, 1.562) -> (-47.182, 6.562)
  line L68 (-47.182, 6.562) -> (-42.182, 6.562)
  line L69 (-42.182, 6.562) -> (-42.182, 1.562)
  line L70 (-42.182, 9.686) -> (-47.182, 9.686)
  line L71 (-47.182, 9.686) -> (-47.182, 14.686)
  line L72 (-47.182, 14.686) -> (-42.182, 14.686)
  line L73 (-42.182, 14.686) -> (-42.182, 9.686)
  line L74 (-42.182, 17.81) -> (-47.182, 17.81)
  line L75 (-47.182, 17.81) -> (-47.182, 22.81)
  line L76 (-47.182, 22.81) -> (-42.182, 22.81)
  line L77 (-42.182, 22.81) -> (-42.182, 17.81)
  line L78 (-42.182, 25.934) -> (-47.182, 25.934)
  line L79 (-47.182, 25.934) -> (-47.182, 30.934)
  line L80 (-47.182, 30.934) -> (-42.182, 30.934)
  line L81 (-42.182, 30.934) -> (-42.182, 25.934)
  line L82 (-42.182, 34.058) -> (-47.182, 34.058)
  line L83 (-47.182, 34.058) -> (-47.182, 39.058)
  line L84 (-47.182, 39.058) -> (-42.182, 39.058)
  line L85 (-42.182, 39.058) -> (-42.182, 34.058)
  line L86 (-42.182, 42.182) -> (-47.182, 42.182)
  line L87 (-47.182, 42.182) -> (-47.182, 47.182)
  line L88 (-47.182, 47.182) -> (-42.182, 47.182)
  line L89 (-42.182, 47.182) -> (-42.182, 42.182)
  line L90 (-42.182, 50.306) -> (-47.182, 50.306)
  line L91 (-47.182, 50.306) -> (-47.182, 55.306)
  line L92 (-47.182, 55.306) -> (-42.182, 55.306)
  line L93 (-42.182, 55.306) -> (-42.182, 50.306)
  line L94 (-42.182, 58.43) -> (-47.182, 58.43)
  line L95 (-47.182, 58.43) -> (-47.182, 63.43)
  line L96 (-47.182, 63.43) -> (-42.182, 63.43)
  line L97 (-42.182, 63.43) -> (-42.182, 58.43)
  line L98 (-34.058, 1.562) -> (-39.058, 1.562)
  line L99 (-39.058, 1.562) -> (-39.058, 6.562)
  line L100 (-39.058, 6.562) -> (-34.058, 6.562)
  line L101 (-34.058, 6.562) -> (-34.058, 1.562)
  line L102 (-34.058, 9.686) -> (-39.058, 9.686)
  line L103 (-39.058, 9.686) -> (-39.058, 14.686)
  line L104 (-39.058, 14.686) -> (-34.058, 14.686)
  line L105 (-34.058, 14.686) -> (-34.058, 9.686)
  line L106 (-34.058, 17.81) -> (-39.058, 17.81)
  line L107 (-39.058, 17.81) -> (-39.058, 22.81)
  line L108 (-39.058, 22.81) -> (-34.058, 22.81)
  line L109 (-34.058, 22.81) -> (-34.058, 17.81)
  line L110 (-34.058, 25.934) -> (-39.058, 25.934)
  line L111 (-39.058, 25.934) -> (-39.058, 30.934)
  line L112 (-39.058, 30.934) -> (-34.058, 30.934)
  line L113 (-34.058, 30.934) -> (-34.058, 25.934)
  line L114 (-34.058, 34.058) -> (-39.058, 34.058)
  line L115 (-39.058, 34.058) -> (-39.058, 39.058)
  line L116 (-39.058, 39.058) -> (-34.058, 39.058)
  line L117 (-34.058, 39.058) -> (-34.058, 34.058)
  line L118 (-34.058, 42.182) -> (-39.058, 42.182)
  line L119 (-39.058, 42.182) -> (-39.058, 47.182)
  line L120 (-39.058, 47.182) -> (-34.058, 47.182)
  line L121 (-34.058, 47.182) -> (-34.058, 42.182)
  line L122 (-34.058, 50.306) -> (-39.058, 50.306)
  line L123 (-39.058, 50.306) -> (-39.058, 55.306)
  line L124 (-39.058, 55.306) -> (-34.058, 55.306)
  line L125 (-34.058, 55.306) -> (-34.058, 50.306)
  line L126 (-34.058, 58.43) -> (-39.058, 58.43)
  line L127 (-39.058, 58.43) -> (-39.058, 63.43)
  line L128 (-39.058, 63.43) -> (-34.058, 63.43)
  line L129 (-34.058, 63.43) -> (-34.058, 58.43)
  line L130 (-25.934, 1.562) -> (-30.934, 1.562)
  line L131 (-30.934, 1.562) -> (-30.934, 6.562)
  line L132 (-30.934, 6.562) -> (-25.934, 6.562)
  line L133 (-25.934, 6.562) -> (-25.934, 1.562)
  line L134 (-25.934, 9.686) -> (-30.934, 9.686)
  line L135 (-30.934, 9.686) -> (-30.934, 14.686)
  line L136 (-30.934, 14.686) -> (-25.934, 14.686)
  line L137 (-25.934, 14.686) -> (-25.934, 9.686)
  line L138 (-25.934, 17.81) -> (-30.934, 17.81)
  line L139 (-30.934, 17.81) -> (-30.934, 22.81)
  line L140 (-30.934, 22.81) -> (-25.934, 22.81)
  line L141 (-25.934, 22.81) -> (-25.934, 17.81)
  line L142 (-25.934, 25.934) -> (-30.934, 25.934)
  line L143 (-30.934, 25.934) -> (-30.934, 30.934)
  line L144 (-30.934, 30.934) -> (-25.934, 30.934)
  line L145 (-25.934, 30.934) -> (-25.934, 25.934)
  line L146 (-25.934, 34.058) -> (-30.934, 34.058)
  line L147 (-30.934, 34.058) -> (-30.934, 39.058)
  line L148 (-30.934, 39.058) -> (-25.934, 39.058)
  line L149 (-25.934, 39.058) -> (-25.934, 34.058)
  line L150 (-25.934, 42.182) -> (-30.934, 42.182)
  line L151 (-30.934, 42.182) -> (-30.934, 47.182)
  line L152 (-30.934, 47.182) -> (-25.934, 47.182)
  line L153 (-25.934, 47.182) -> (-25.934, 42.182)
  line L154 (-25.934, 50.306) -> (-30.934, 50.306)
  line L155 (-30.934, 50.306) -> (-30.934, 55.306)
  line L156 (-30.934, 55.306) -> (-25.934, 55.306)
  line L157 (-25.934, 55.306) -> (-25.934, 50.306)
  line L158 (-25.934, 58.43) -> (-30.934, 58.43)
  line L159 (-30.934, 58.43) -> (-30.934, 63.43)
  line L160 (-30.934, 63.43) -> (-25.934, 63.43)
  line L161 (-25.934, 63.43) -> (-25.934, 58.43)
  line L162 (-17.81, 1.562) -> (-22.81, 1.562)
  line L163 (-22.81, 1.562) -> (-22.81, 6.562)
  line L164 (-22.81, 6.562) -> (-17.81, 6.562)
  line L165 (-17.81, 6.562) -> (-17.81, 1.562)
  line L166 (-17.81, 9.686) -> (-22.81, 9.686)
  line L167 (-22.81, 9.686) -> (-22.81, 14.686)
  line L168 (-22.81, 14.686) -> (-17.81, 14.686)
  line L169 (-17.81, 14.686) -> (-17.81, 9.686)
  line L170 (-17.81, 17.81) -> (-22.81, 17.81)
  line L171 (-22.81, 17.81) -> (-22.81, 22.81)
  line L172 (-22.81, 22.81) -> (-17.81, 22.81)
  line L173 (-17.81, 22.81) -> (-17.81, 17.81)
  line L174 (-17.81, 25.934) -> (-22.81, 25.934)
  line L175 (-22.81, 25.934) -> (-22.81, 30.934)
  line L176 (-22.81, 30.934) -> (-17.81, 30.934)
  line L177 (-17.81, 30.934) -> (-17.81, 25.934)
  line L178 (-17.81, 34.058) -> (-22.81, 34.058)
  line L179 (-22.81, 34.058) -> (-22.81, 39.058)
  line L180 (-22.81, 39.058) -> (-17.81, 39.058)
  line L181 (-17.81, 39.058) -> (-17.81, 34.058)
  line L182 (-17.81, 42.182) -> (-22.81, 42.182)
  line L183 (-22.81, 42.182) -> (-22.81, 47.182)
  line L184 (-22.81, 47.182) -> (-17.81, 47.182)
  line L185 (-17.81, 47.182) -> (-17.81, 42.182)
  line L186 (-17.81, 50.306) -> (-22.81, 50.306)
  line L187 (-22.81, 50.306) -> (-22.81, 55.306)
  line L188 (-22.81, 55.306) -> (-17.81, 55.306)
  line L189 (-17.81, 55.306) -> (-17.81, 50.306)
  line L190 (-17.81, 58.43) -> (-22.81, 58.43)
  line L191 (-22.81, 58.43) -> (-22.81, 63.43)
  line L192 (-22.81, 63.43) -> (-17.81, 63.43)
  line L193 (-17.81, 63.43) -> (-17.81, 58.43)
  line L194 (-9.686, 1.562) -> (-14.686, 1.562)
  line L195 (-14.686, 1.562) -> (-14.686, 6.562)
  line L196 (-14.686, 6.562) -> (-9.686, 6.562)
  line L197 (-9.686, 6.562) -> (-9.686, 1.562)
  line L198 (-9.686, 9.686) -> (-14.686, 9.686)
  line L199 (-14.686, 9.686) -> (-14.686, 14.686)
  line L200 (-14.686, 14.686) -> (-9.686, 14.686)
  line L201 (-9.686, 14.686) -> (-9.686, 9.686)
  line L202 (-9.686, 17.81) -> (-14.686, 17.81)
  line L203 (-14.686, 17.81) -> (-14.686, 22.81)
  line L204 (-14.686, 22.81) -> (-9.686, 22.81)
  line L205 (-9.686, 22.81) -> (-9.686, 17.81)
  line L206 (-9.686, 25.934) -> (-14.686, 25.934)
  line L207 (-14.686, 25.934) -> (-14.686, 30.934)
  line L208 (-14.686, 30.934) -> (-9.686, 30.934)
  line L209 (-9.686, 30.934) -> (-9.686, 25.934)
  line L210 (-9.686, 34.058) -> (-14.686, 34.058)
  line L211 (-14.686, 34.058) -> (-14.686, 39.058)
  line L212 (-14.686, 39.058) -> (-9.686, 39.058)
  line L213 (-9.686, 39.058) -> (-9.686, 34.058)
  line L214 (-9.686, 42.182) -> (-14.686, 42.182)
  line L215 (-14.686, 42.182) -> (-14.686, 47.182)
  line L216 (-14.686, 47.182) -> (-9.686, 47.182)
  line L217 (-9.686, 47.182) -> (-9.686, 42.182)
  line L218 (-9.686, 50.306) -> (-14.686, 50.306)
  line L219 (-14.686, 50.306) -> (-14.686, 55.306)
  line L220 (-14.686, 55.306) -> (-9.686, 55.306)
  line L221 (-9.686, 55.306) -> (-9.686, 50.306)
  line L222 (-9.686, 58.43) -> (-14.686, 58.43)
  line L223 (-14.686, 58.43) -> (-14.686, 63.43)
  line L224 (-14.686, 63.43) -> (-9.686, 63.43)
  line L225 (-9.686, 63.43) -> (-9.686, 58.43)
  line L226 (-1.562, 1.562) -> (-6.562, 1.562)
  line L227 (-6.562, 1.562) -> (-6.562, 6.562)
  line L228 (-6.562, 6.562) -> (-1.562, 6.562)
  line L229 (-1.562, 6.562) -> (-1.562, 1.562)
  line L230 (-1.562, 9.686) -> (-6.562, 9.686)
  line L231 (-6.562, 9.686) -> (-6.562, 14.686)
  line L232 (-6.562, 14.686) -> (-1.562, 14.686)
  line L233 (-1.562, 14.686) -> (-1.562, 9.686)
  line L234 (-1.562, 17.81) -> (-6.562, 17.81)
  line L235 (-6.562, 17.81) -> (-6.562, 22.81)
  line L236 (-6.562, 22.81) -> (-1.562, 22.81)
  line L237 (-1.562, 22.81) -> (-1.562, 17.81)
  line L238 (-1.562, 25.934) -> (-6.562, 25.934)
  line L239 (-6.562, 25.934) -> (-6.562, 30.934)
  line L240 (-6.562, 30.934) -> (-1.562, 30.934)
  line L241 (-1.562, 30.934) -> (-1.562, 25.934)
  line L242 (-1.562, 34.058) -> (-6.562, 34.058)
  line L243 (-6.562, 34.058) -> (-6.562, 39.058)
  line L244 (-6.562, 39.058) -> (-1.562, 39.058)
  line L245 (-1.562, 39.058) -> (-1.562, 34.058)
  line L246 (-1.562, 42.182) -> (-6.562, 42.182)
  line L247 (-6.562, 42.182) -> (-6.562, 47.182)
  line L248 (-6.562, 47.182) -> (-1.562, 47.182)
  line L249 (-1.562, 47.182) -> (-1.562, 42.182)
  line L250 (-1.562, 50.306) -> (-6.562, 50.306)
  line L251 (-6.562, 50.306) -> (-6.562, 55.306)
  line L252 (-6.562, 55.306) -> (-1.562, 55.306)
  line L253 (-1.562, 55.306) -> (-1.562, 50.306)
  line L254 (-1.562, 58.43) -> (-6.562, 58.43)
  line L255 (-6.562, 58.43) -> (-6.562, 63.43)
  line L256 (-6.562, 63.43) -> (-1.562, 63.43)
  line L257 (-1.562, 63.43) -> (-1.562, 58.43)
  point P0 (0, 0)
  dimension "d79" = 8.124
  dimension "d82" = 8.124
  constraints: 516 end point, 2 collinear, 2 parallel, 1 horizontal, 1 perpendicular, 1 vertical, 503 other
  measures "d79" distance of L2.start L6.start
  measures "d82" distance of L2.start L34.start
extrude "Extrusion6" cut sketch "Sketch3" against normal blind 10
body "Solid1"
